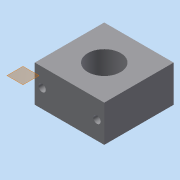
# Autodesk Inventor part: palier_roulement_bras
Saved by Autodesk Inventor 2016 (Build 200138000, 138)
## iProperties
Created: 2016-12-04
Part Number: palier_roulement_bras
Material: Generic
Document SubType Name: Modeling
Designer: Aegir
Density: 1 g/cm^3
Appearance: Default
Author: Aegir
Autodesk Inventor part; units mm, degrees
ref_plane "YZ Plane" through (0, 0, 0) normal (1, 0, 0) x (0, 1, 0)
ref_plane "XZ Plane" through (0, 0, 0) normal (0, 1, 0) x (-1, 0, 0)
ref_plane "XY Plane" through (0, 0, 0) normal (0, 0, 1) x (1, 0, 0)
sketch "Esquisse1" plane through (0, 0, 0) normal (0, 0, 1) x (1, 0, 0)
  line L0 (-73.2723, 18.1488) -> (-54.2723, 18.1488)
  line L1 (-54.2723, 18.1488) -> (-54.2723, 37.1488)
  line L2 (-54.2723, 37.1488) -> (-73.2723, 37.1488)
  line L3 (-73.2723, 37.1488) -> (-73.2723, 18.1488)
  circle A0 centre (-63.7723, 27.6488) radius 4.5
  point P0 (0, 0)
  dimension "d0" = 19
  dimension "d1" = 19
  dimension "d2" = 9
  constraints: 8 end point, 2 parallel, 1 centre point, 1 horizontal, 1 perpendicular
  measures "d0" distance of L2.end L0.start
  measures "d1" distance of L1.end L2.end
  measures "d2" diameter of A0
extrude "Extrusion1" add sketch "Esquisse1" along normal blind 10
sketch "Esquisse2" plane through (-73.2723, 37.1488, 0) normal (0, 1, 0) x (1, 0, 0)
  line L0 (0, 0) -> (0, -10) projected
  line L1 (19, 0) -> (19, -10) projected
  line L2 (19, -10) -> (0, -10) projected
  point P0 (73.2723, 0)
  point P1 (2, -5)
  point P2 (17, -5)
  dimension "d5" = 2
  dimension "d6" = 2
  dimension "d7" = 5
  dimension "d8" = 5
  measures "d5" distance from line of L0 point (2, -5)
  measures "d6" distance from line of L1 point (17, -5)
  measures "d7" distance from line of L2 point (2, -5)
  measures "d8" distance from line of L2 point (17, -5)
hole "Perçage1" at (-71.2723, 37.1488, 5) at (-56.2723, 37.1488, 5) direction (0, -1, 0) diameter 2 end through all
ref_plane "Plan de construction1" through (-63.7723, 27.6488, 10.9) normal (0, 0, 1) x (1, 0, 0)
